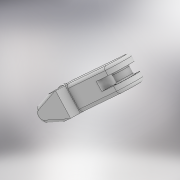
# Autodesk Inventor part: Upper Arm
Saved by Autodesk Inventor 2022 (Build 260153000, 153)
## iProperties
Created: 2022-02-25
Part Number: Upper Arm
Material: Generic
Document SubType Name: Modeling
Designer: joshw
Density: 1 g/cm^3
Appearance: Default
Author: joshw
Autodesk Inventor part; units mm, degrees
ref_plane "YZ Plane" through (0, 0, 0) normal (1, 0, 0) x (0, 1, 0)
ref_plane "XZ Plane" through (0, 0, 0) normal (0, 1, 0) x (-1, 0, 0)
ref_plane "XY Plane" through (0, 0, 0) normal (0, 0, 1) x (1, 0, 0)
sketch "Sketch1" plane through (0, 0, 0) normal (0, 0, 1) x (1, 0, 0)
  circle A0 centre (-13.7753, -14.5826) radius 2.5
  line L0 (-12.5696, -16.7726) -> (-6.7753, -13.5826)
  line L1 (-6.7753, -13.5826) -> (14.7028, 6.1537)
  line L2 (14.7028, 6.1537) -> (13.0113, 7.9946)
  line L3 (13.0113, 7.9946) -> (5.648, 1.2284)
  line L4 (5.648, 1.2284) -> (4.633, 2.3329)
  line L5 (-13.7753, -14.5826) -> (25.6156, 21.6139)
  circle A1 centre (-13.7753, -14.5826) radius 2.5
  line L6 (-15.8558, -13.1964) -> (-12.1883, -7.6919)
  line L7 (-12.1883, -7.6919) -> (9.2899, 12.0444)
  line L8 (9.2899, 12.0444) -> (10.9814, 10.2036)
  line L9 (10.9814, 10.2036) -> (3.6181, 3.4374)
  line L10 (3.6181, 3.4374) -> (4.633, 2.3329)
  circle A2 centre (-13.7753, -14.5826) radius 7.0711
  point P0 (0, 0)
  point P1 (0, 0)
  point P2 (1.9176, -2.0868)
  point P3 (1.9176, -2.0868)
  point P4 (-15.4817, 12.292)
  dimension "d4" = 5
  dimension "d1" = 2.5
  dimension "d3" = 1.5
  dimension "d6" = 7
  dimension "d7" = 1
  dimension "d8" = 35
  dimension "d9" = 10
  constraints: 22 end point, 7 symmetric about line, 4 perpendicular, 1 coincident, 1 point on line, 11 other
  measures "d1" distance between parallel lines of L1 L3
  measures "d3" distance of L4.end L3.end
  measures "d6" horizontal distance of L0.end L5.start
  measures "d7" vertical distance of L0.end L5.start
  measures "d8" distance from line of L2 L5.start
  measures "d9" distance between parallel lines of L2 L4
extrude "Extrusion1" add sketch "Sketch1" along normal blind 8.5 contours L7 L8 L9 L10 L5 A2 | A2 L5 L4 L3 L2 L1
sketch "Sketch2" plane through (-12.1883, -7.6919, 8.5) normal (-0.676619, 0.7363333, 0) x (0.7363333, 0.676619, 0)
  line L0 (29.169, 8.5) -> (0, 8.5) projected
  line L1 (0, 8.5) -> (0, 0) projected
  line L2 (29.169, 0) -> (0, 0) projected
  line L3 (29.169, 8.5) -> (29.169, 0) projected
  circle A0 centre (24.919, 4.25) radius 4.25
  point P0 (14.1791, 8.5)
  point P1 (24.919, 8.5)
  point P2 (29.169, 4.25)
  point P3 (24.919, 0)
  constraints: 3 tangent, 1 centre point
extrude "Extrusion2" cut sketch "Sketch2" against normal blind 12.5 contours L3 A0 L0 | L3 L2 A0
sketch "Sketch3" plane through (-12.1883, -7.6919, 8.5) normal (-0.676619, 0.7363333, 0) x (0.7363333, 0.676619, 0)
  line L0 (6.5908, 0.2398) -> (-11.4092, 0.2398)
  line L1 (-11.4092, 0.2398) -> (-11.4092, -2.2602)
  line L2 (-11.4092, -2.2602) -> (6.5908, -2.2602)
  line L3 (6.5908, -2.2602) -> (6.5908, 0.2398)
  point P0 (14.1791, 8.5)
  dimension "d14" = 18
  dimension "d15" = 2.5
  constraints: 8 end point, 2 parallel, 1 horizontal, 1 perpendicular
  measures "d14" distance of L2.end L1.end
  measures "d15" distance of L1.end L0.end
extrude "Extrusion3" add sketch "Sketch3" against normal up to surface (8 mm away)
extrude "Extrusion4" cut sketch "Sketch1" along normal blind 35.25 contours A0 L0 A2 L6
sketch "Sketch4" plane through (-13.7753, -14.5826, 8.2602) normal (0, 0, -1) x (-0.7363333, -0.676619, 0)
  arc A0 (0.594, -2.4284) -> (0.594, 2.4284) centre (0, 0) ccw projected
  circle A1 centre (0, 0) radius 2.5
  point P0 (-20.0101, 1.417)
  point P1 (0.594, 2.4284)
  point P2 (0.594, -2.4284)
  constraints: 1 centre point, 1 coincident
extrude "Extrusion5" add sketch "Sketch4" along normal blind 7
sketch "Sketch5" plane through (-13.7753, -14.5826, 1.2602) normal (0, 0, -1) x (-1, 0, 0)
  circle A0 centre (0, 0) radius 2.5 projected
  circle A1 centre (0, 0) radius 4.05
  point P0 (-13.7753, 14.5826)
  dimension "d22" = 8.1
  constraints: 1 centre point, 1 coincident
  measures "d22" diameter of A1
extrude "Extrusion6" add sketch "Sketch5" along normal up to surface (1.2602 mm away) contours A0 | A1
chamfer "Chamfer1" distance 2 angle 45 1 edges at (-4.6288, -6.1778, 10.7602)
fillet "Fillet1" radius 1 9 edges at (-15.6161, -16.2742, 10.7602) (-14.022, -10.4442, 10.7602) (-9.6724, -15.1776, 10.7602) (14.7028, 6.1537, 4.25) (2.3991, -5.1523, 0) (4.8256, -2.9225, 8.5) (9.2899, 12.0444, 4.25) (-3.0139, 0.7384, 0) (-0.5874, 2.9681, 8.5)
sketch "Sketch6" plane through (5.648, 1.2284, 8.5) normal (-0.676619, 0.7363333, 0) x (0.7363333, 0.676619, 0)
  arc A0 (5.75, 0) -> (5.75, 8.5) centre (5.75, 4.25) ccw projected
  circle A1 centre (5.75, 4.25) radius 2.5
  point P0 (-4.9899, 8.5)
  dimension "d29" = 5
  constraints: 1 centre point, 1 coincident
  measures "d29" diameter of A1
extrude "Extrusion7" add sketch "Sketch6" along normal up to surface (3 mm away)
ref_plane "Work Plane1" through (8.8669, 6.2234, 4.25) normal (0.676619, -0.7363333, 0) x (0.7363333, 0.676619, 0)
fillet "Fillet2" radius 0.5 1 edges at (-11.9345, -12.8911, 8.2602)
chamfer "Chamfer2" distance 1 angle 45 1 edges at (-8.5686, -9.7982, 8.2602)
fillet "Fillet3" radius 0.5 2 edges at (8.041, 3.4274, 4.25) (6.0112, 5.6364, 4.25)
body "Solid1"
